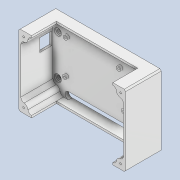
# Autodesk Inventor part: 10-06-009
Saved by Autodesk Inventor 2020 (Build 240168000, 168)
## iProperties
Created: 2019-11-09
Part Number: 10-06-009
Material: ABS Plastic
Document SubType Name: Modeling
Designer: iuliu
Density: 1.06 g/cm^3
Appearance: Smooth - White
Mass: 128.602 g
Surface Area: 588.497 cm^2
Volume: 121.322 cm^3
Description: Cutie Arduino
Author: iuliu
Subject: 027
Autodesk Inventor part; units mm, degrees
ref_plane "YZ Plane" through (0, 0, 0) normal (1, 0, 0) x (0, 1, 0)
ref_plane "XZ Plane" through (0, 0, 0) normal (0, 1, 0) x (-1, 0, 0)
ref_plane "XY Plane" through (0, 0, 0) normal (0, 0, 1) x (1, 0, 0)
sketch "Sketch1" plane through (0, 0, 0) normal (0, 0, 1) x (1, 0, 0)
  line L0 (-75, 50) -> (75, 50)
  line L1 (75, 50) -> (75, -50)
  line L2 (75, -50) -> (-75, -50)
  line L3 (-75, -50) -> (-75, 50)
  point P0 (0, 0)
  point P1 (-75, 0)
  point P2 (0, 50)
  dimension "d0" = 150
  dimension "d1" = 100
  constraints: 8 end point, 2 midpoint, 2 parallel, 1 horizontal, 1 horizontal alignment, 1 perpendicular, 1 vertical alignment
  measures "d0" distance of L0.start L0.end
  measures "d1" distance of L2.end L0.start
extrude "Extrusion1" add sketch "Sketch1" along normal blind 50
sketch "Sketch2" plane through (0, 0, 50) normal (0, 0, 1) x (1, 0, 0)
  line L0 (-33.0476, 12.9868) -> (-30.2047, 12.9868) construction
  line L1 (-30.2047, 12.9868) -> (-30.2047, 9.9388) construction
  line L2 (-30.2047, 9.9388) -> (-33.0476, 9.9388) construction
  line L3 (-33.0476, 9.9388) -> (-33.0476, 12.9868) construction
  point P0 (0, 0)
  constraints: 2 other
sketch "Sketch3" plane through (0, 0, 50) normal (0, 0, 1) x (1, 0, 0)
  line L0 (75, -50) -> (75, 50) projected
  line L1 (75, 50) -> (-75, 50) projected
  line L2 (-75, 50) -> (-75, -50) projected
  line L3 (-75, -50) -> (75, -50) projected
  line L4 (-72, 47) -> (72, 47)
  line L5 (72, 47) -> (72, -47)
  line L6 (72, -47) -> (-72, -47)
  line L7 (-72, -47) -> (-72, 47)
  point P0 (0, 0)
  dimension "d4" = 3
  constraints: 8 end point, 3 other
  measures "d4" distance between parallel lines of L1 L4
extrude "Extrusion2" cut sketch "Sketch3" against normal blind 45 contours L4 L5 L6 L7
sketch "Sketch4" plane through (-75, -50, 0) normal (-1, 0, 0) x (0, 0, 1)
  line L0 (26.325, 30.96) -> (27.325, 30.96) construction
  line L1 (27.325, 30.96) -> (27.325, 29.96) construction
  line L2 (27.325, 29.96) -> (26.325, 29.96) construction
  line L3 (26.325, 29.96) -> (26.325, 30.96) construction
  line L4 (21, 20) -> (21, 81.7649) construction
  line L5 (21, 81.7649) -> (23, 81.7649) construction
  line L6 (23, 81.7649) -> (23, 44.32) construction
  line L7 (23, 44.32) -> (31.5, 44.32) construction
  line L8 (31.5, 44.32) -> (31.5, 44.16) construction
  line L9 (31.5, 44.16) -> (31.1, 44.16) construction
  line L10 (31.1, 44.16) -> (31.1, 22) construction
  line L11 (31.1, 22) -> (23, 22) construction
  line L12 (23, 22) -> (23, 20) construction
  line L13 (23, 20) -> (21, 20) construction
  line L14 (6.5168, 74.0273) -> (6.48, 74.0735) construction
  line L15 (6.48, 74.0735) -> (6.48, 74.4839) construction
  line L16 (6.48, 74.4839) -> (7.0709, 74.9548) construction
  arc A0 (8, 75.2183) -> (7.0709, 74.9548) centre (7.85, 73.9773) ccw construction
  line L17 (8, 75.2183) -> (8, 81.2973) construction
  line L18 (8, 81.2973) -> (10, 81.2973) construction
  line L19 (10, 81.2973) -> (10, 73.7973) construction
  line L20 (10, 73.7973) -> (20.5, 73.7973) construction
  line L21 (20.5, 73.7973) -> (20.5, 61.7973) construction
  line L22 (20.5, 61.7973) -> (10, 61.7973) construction
  line L23 (10, 61.7973) -> (10, 43.2973) construction
  line L24 (10, 43.2973) -> (16.35, 43.2973) construction
  line L25 (16.35, 43.2973) -> (16.35, 42.7893) construction
  arc A1 (16.35, 34.6613) -> (16.35, 42.7893) centre (16.35, 38.7253) ccw construction
  line L26 (16.35, 34.6613) -> (16.35, 34.1533) construction
  line L27 (16.35, 34.1533) -> (10, 34.1533) construction
  line L28 (10, 34.1533) -> (10, 28.1327) construction
  line L29 (10, 28.1327) -> (8, 28.1327) construction
  line L30 (8, 28.1327) -> (8, 60.3763) construction
  arc A2 (7.0709, 60.6398) -> (8, 60.3763) centre (7.85, 61.6173) ccw construction
  line L31 (7.0709, 60.6398) -> (6.48, 61.1107) construction
  line L32 (6.48, 61.1107) -> (6.48, 61.5211) construction
  line L33 (6.48, 61.5211) -> (6.5168, 61.5673) construction
  line L34 (6.5168, 61.5673) -> (7.3078, 60.9369) construction
  arc A3 (7.3078, 60.9369) -> (8, 60.7603) centre (7.85, 61.6173) ccw construction
  line L35 (8, 60.7603) -> (8, 74.8343) construction
  arc A4 (8, 74.8343) -> (7.3078, 74.6577) centre (7.85, 73.9773) ccw construction
  line L36 (7.3078, 74.6577) -> (6.5168, 74.0273) construction
  circle A5 centre (16.35, 38.7253) radius 3.048 construction
  circle A6 centre (16.35, 38.7253) radius 1 construction
  line L37 (27.325, 41.12) -> (27.325, 40.12) construction
  line L38 (27.325, 40.12) -> (26.325, 40.12) construction
  line L39 (26.325, 40.12) -> (26.325, 41.12) construction
  line L40 (26.325, 41.12) -> (27.325, 41.12) construction
  arc A7 (24.7, 32.705) -> (24.7, 28.215) centre (27.05, 30.46) ccw construction
  line L41 (24.7, 28.215) -> (24.7, 27.625) construction
  arc A8 (24.7, 27.625) -> (24.7, 23.135) centre (27.05, 25.38) ccw construction
  line L42 (24.7, 23.135) -> (24.7, 22.78) construction
  line L43 (24.7, 22.78) -> (30.05, 22.78) construction
  line L44 (30.05, 22.78) -> (30.05, 43.22) construction
  line L45 (30.05, 43.22) -> (24.7, 43.22) construction
  line L46 (24.7, 43.22) -> (24.7, 42.865) construction
  arc A9 (24.7, 42.865) -> (24.7, 38.375) centre (27.05, 40.62) ccw construction
  line L47 (24.7, 38.375) -> (24.7, 37.785) construction
  arc A10 (24.7, 37.785) -> (24.7, 33.295) centre (27.05, 35.54) ccw construction
  line L48 (24.7, 33.295) -> (24.7, 32.705) construction
  line L49 (26.325, 24.88) -> (26.325, 25.88) construction
  line L50 (26.325, 25.88) -> (27.325, 25.88) construction
  line L51 (27.325, 25.88) -> (27.325, 24.88) construction
  line L52 (27.325, 24.88) -> (26.325, 24.88) construction
  line L53 (26.325, 35.04) -> (26.325, 36.04) construction
  line L54 (26.325, 36.04) -> (27.325, 36.04) construction
  line L55 (27.325, 36.04) -> (27.325, 35.04) construction
  line L56 (27.325, 35.04) -> (26.325, 35.04) construction
  line L57 (34.1, 47.32) -> (18, 47.32)
  line L58 (18, 47.32) -> (18, 17)
  line L59 (18, 17) -> (34.1, 17)
  line L60 (34.1, 17) -> (34.1, 47.32)
  line L61 (23.5, 76.7973) -> (7, 76.7973)
  line L62 (7, 76.7973) -> (7, 58.7973)
  line L63 (7, 58.7973) -> (23.5, 58.7973)
  line L64 (23.5, 58.7973) -> (23.5, 76.7973)
  point P0 (0, 50)
  dimension "d9" = 3
  dimension "d10" = 3
  dimension "d11" = 3
  dimension "d12" = 3
  dimension "d13" = 3
  dimension "d14" = 3
  dimension "d16" = 3
  dimension "d17" = 3
  constraints: 130 end point, 26 vertical, 23 horizontal, 18 point on circle, 11 centre point, 4 parallel, 2 perpendicular, 98 other
  measures "d9" distance from line of L10.end L60
  measures "d10" distance from line of L4.start L59
  measures "d11" distance from line of L6.end L57
  measures "d12" distance from line of L58 L4.start
  measures "d13" distance from line of L21.end L64
  measures "d14" distance from line of L22.end L63
  measures "d16" distance from line of L19.end L61
  measures "d17" distance from line of L62 L19.end
extrude "Extrusion3" cut sketch "Sketch4" against normal up to surface (3 mm away) contours L64 L63 L62 L61
sketch "Sketch5" plane through (-75, 50, 0) normal (0, 1, 0) x (1, 0, 0)
  circle A0 centre (112.5, -25) radius 7.5
  circle A1 centre (37.5, -25) radius 7.5
  circle A2 centre (75, -25) radius 7.5
  line L0 (150, 0) -> (150, -50) projected
  line L1 (0, 0) -> (0, -50) projected
  point P0 (75, 0)
  point P1 (0, -25)
  point P2 (0, -25)
  dimension "d20" = 15
  dimension "d21" = 15
  dimension "d22" = 15
  dimension "d23" = 37.5
  dimension "d24" = 37.5
  dimension "d25" = 37.5
  constraints: 3 centre point, 3 horizontal alignment, 2 midpoint
  measures "d20" diameter of A0
  measures "d21" diameter of A1
  measures "d22" diameter of A2
  measures "d23" distance from line of L0 A0.centre
  measures "d24" distance of A2.centre A0.centre
  measures "d25" distance of A2.centre A1.centre
extrude "Extrusion4" [suppressed]
sketch "Sketch6" plane through (0, 0, 5) normal (0, 0, 1) x (1, 0, 0)
  line L0 (-68, -43) -> (68, -43) construction
  line L1 (68, -43) -> (68, 43) construction
  line L2 (68, 43) -> (-68, 43) construction
  line L3 (-68, 43) -> (-68, -43) construction
  line L4 (-72, -47) -> (-72, 47) projected
  line L5 (-72, 47) -> (72, 47) projected
  line L6 (72, 47) -> (72, -47) projected
  line L7 (72, -47) -> (-72, -47) projected
  point P0 (0, 0)
  dimension "d28" = 4
  dimension "d29" = 4
  dimension "d30" = 4
  dimension "d31" = 4
  constraints: 8 end point, 2 parallel, 1 horizontal, 1 perpendicular
  measures "d28" distance between parallel lines of L3 L4
  measures "d29" distance between parallel lines of L5 L2
  measures "d30" distance between parallel lines of L6 L1
  measures "d31" distance between parallel lines of L7 L0
hole "Hole1" at (-68, -43, 5) at (-68, 43, 5) at (68, -43, 5) at (68, 43, 5) direction (0, 0, -1) diameter 2.5 end through all
sketch "Sketch7" plane through (0, 0, 5) normal (0, 0, 1) x (1, 0, 0)
  circle A0 centre (-68, -43) radius 1.25 projected
  circle A1 centre (-68, 43) radius 1.25 projected
  circle A2 centre (68, 43) radius 1.25 projected
  circle A3 centre (68, -43) radius 1.25 projected
  circle A4 centre (-68, -43) radius 6
  circle A5 centre (-68, 43) radius 6
  circle A6 centre (68, -43) radius 6
  circle A7 centre (68, 43) radius 6
  point P0 (0, 0)
  dimension "d39" = 12
  constraints: 4 centre point, 4 coincident, 3 equal radius
  measures "d39" diameter of A4
extrude "Extrusion5" add sketch "Sketch7" along normal up to surface (45 mm away)
fillet "Fillet1" radius 5 8 edges at (-72, 38.5279, 27.5) (-63.5279, 47, 27.5) (-63.5279, -47, 27.5) (-72, -38.5279, 27.5) (63.5279, 47, 27.5) (63.5279, -47, 27.5) (72, 38.5279, 27.5) (72, -38.5279, 27.5)
sketch "Sketch10" plane through (0, 0, 0) normal (0, 0, -1) x (-1, 0, 0)
  line L0 (-75, 50) -> (-55, 50)
  line L1 (-55, 50) -> (-55, -50)
  line L2 (-55, -50) -> (-75, -50)
  line L3 (-75, -50) -> (-75, 50)
  line L4 (-75, 50) -> (75, 50) projected
  line L5 (75, -50) -> (-75, -50) projected
  line L6 (-75, -50) -> (-75, 50) projected
  point P0 (0, 0)
  dimension "d46" = 20
  constraints: 8 end point, 3 collinear, 2 parallel, 1 horizontal, 1 perpendicular
  measures "d46" distance of L0.start L0.end
extrude "Extrusion7" [suppressed]
sketch "Sketch11" plane through (0, 0, 5) normal (0, 0, 1) x (1, 0, 0)
  line L0 (72, 32.0455) -> (72, -32.0455) projected
  line L1 (57.0455, -47) -> (-57.0455, -47) projected
  line L2 (75, 50) -> (-75, 50) projected
  point P0 (0, 0)
  point P1 (65, -17)
  point P2 (65, 20)
  dimension "d49" = 7
  dimension "d50" = 30
  dimension "d51" = 30
  constraints: 1 vertical alignment
  measures "d49" distance from line of L0 point (65, -17)
  measures "d50" distance from line of L1 point (65, -17)
  measures "d51" distance from line of L2 point (65, 20)
hole "Hole2" at (65, -17, 5) at (65, 20, 5) direction (0, 0, -1) diameter 7 end through all
sketch "Sketch12" plane through (0, 0, 5) normal (0, 0, 1) x (1, 0, 0)
  line L0 (-50, -42) -> (50, -42) construction
  line L1 (-50, -47) -> (50, -47)
  line L2 (50, -37) -> (-50, -37)
  arc A0 (-50, -37) -> (-50, -47) centre (-50, -42) ccw
  arc A1 (50, -47) -> (50, -37) centre (50, -42) ccw
  line L3 (-66.4643, 0) -> (-31.6341, 0) construction
  line L4 (57.0455, -47) -> (-57.0455, -47) construction
  line L5 (-50, 47) -> (50, 47)
  line L6 (50, 37) -> (-50, 37)
  arc A2 (-50, 47) -> (-50, 37) centre (-50, 42) ccw
  arc A3 (50, 37) -> (50, 47) centre (50, 42) ccw
  point P0 (0, 0)
  point P1 (0, -42)
  point P2 (-49.0492, 0)
  dimension "d59" = 10
  dimension "d60" = 5
  dimension "d61" = 100
  constraints: 14 end point, 8 point on circle, 6 symmetric about line, 4 centre point, 4 tangent, 2 horizontal, 2 midpoint, 1 horizontal alignment, 1 parallel, 1 vertical alignment, 2 other
  measures "d59" distance between parallel lines of L2 L1
  measures "d60" distance between parallel lines of L4 L0
  measures "d61" distance of L0.start L0.end
extrude "Extrusion8" cut sketch "Sketch12" against normal through all
sketch "Sketch13" plane through (0, 0, 5) normal (0, 0, 1) x (1, 0, 0)
  circle A0 centre (-53, -19.3673) radius 1.6078 construction
  circle A1 centre (-51.7238, 29.1287) radius 1.6078 construction
  circle A2 centre (22.9611, 28.7987) radius 1.6 construction
  circle A3 centre (29.9537, -19.3673) radius 1.6078 construction
  circle A4 centre (-63.3989, 10.0987) radius 1.1 construction
  point P0 (0, 0)
hole "Hole3" at (-53, -19.3673, 5) at (-51.7238, 29.1287, 5) at (29.9537, -19.3673, 5) at (22.9611, 28.7987, 5) direction (0, 0, -1) diameter 2.459 end through all thread size "M3x0.5" class "6H" standard "ISO Metric profile"
chamfer "Chamfer1" distance 2 angle 45 4 edges at (-53, -18.1378, 0) (29.9537, -18.1378, 0) (-51.7238, 30.3582, 0) (22.9611, 30.0282, 0)
sketch "Sketch14" plane through (0, 0, 5) normal (0, 0, 1) x (1, 0, 0)
  circle A0 centre (-68, -43) radius 1.25 projected
  circle A1 centre (-68, 43) radius 1.25 projected
  line L0 (-75, 50) -> (-75, -50) projected
  point P0 (0, 0)
  point P1 (-65, -28)
  point P2 (-65, 28)
  dimension "d74" = 15
  dimension "d75" = 15
  dimension "d83" = 10
  constraints: 1 vertical alignment
  measures "d74" vertical distance of A0.centre point (-65, -28)
  measures "d75" vertical distance of A1.centre point (-65, 28)
  measures "d83" distance from line of point (-65, -28) L0
hole "Hole4" at (-65, -28, 5) at (-65, 28, 5) direction (0, 0, -1) diameter 5 end through all counterbore diameter 10 counterbore depth 2
sketch "Sketch15" plane through (-75, 50, 50) normal (0, 1, 0) x (1, 0, 0)
  line L0 (125, 5) -> (25, 5) construction
  line L1 (125, 3.5) -> (25, 3.5)
  line L2 (25, 6.5) -> (125, 6.5)
  arc A0 (125, 3.5) -> (125, 6.5) centre (125, 5) ccw
  arc A1 (25, 6.5) -> (25, 3.5) centre (25, 5) ccw
  line L3 (0, 50) -> (0, 0) projected
  line L4 (150, 50) -> (150, 0) projected
  line L5 (150, 0) -> (0, 0) projected
  point P0 (75, 50)
  point P1 (75, 5)
  point P2 (150, 70)
  dimension "d84" = 3
  dimension "d85" = 25
  dimension "d86" = 25
  dimension "d87" = 5
  constraints: 8 end point, 4 point on circle, 4 tangent, 2 centre point, 1 horizontal, 1 midpoint, 1 parallel
  measures "d84" distance between parallel lines of L2 L1
  measures "d85" distance from line of L3 L0.end
  measures "d86" distance from line of L4 L0.start
  measures "d87" distance between parallel lines of L0 L5
extrude "Extrusion9" [suppressed]
pattern_linear "Rectangular Pattern1" [suppressed]
sketch "Sketch16" plane through (0, 0, 0) normal (0, 1, 0) x (-1, 0, 0)
  line L0 (57.0455, 50) -> (57.0455, 5) projected
  line L1 (-57.0455, 5) -> (-57.0455, 50) projected
  line L2 (50, 5) -> (-50, 5) projected
  line L3 (-57.0455, 50) -> (-57.0455, 5) projected
  line L4 (-57.0455, 15) -> (57.0455, 15)
  line L5 (57.0455, 5) -> (57.0455, 50) projected
  line L6 (-57.0455, 50) -> (57.0455, 50)
  line L7 (75, 50) -> (-75, 50) projected
  point P0 (0, 0)
  dimension "d93" = 10
  constraints: 4 end point, 2 point on line, 1 collinear, 1 perpendicular
  measures "d93" distance between parallel lines of L2 L4
extrude "Extrusion10" cut sketch "Sketch16" against normal through all both and the other way through all
chamfer "Chamfer2" distance 2 angle 45 4 edges at (75, 50, 25) (-75, 50, 25) (-75, -50, 25) (75, -50, 25)
sketch "Sketch17" plane through (0, 0, 5) normal (0, 0, 1) x (1, 0, 0)
  circle A0 centre (-65, -28) radius 5 projected
  circle A1 centre (-65, 28) radius 5 projected
  circle A2 centre (29.9537, -19.3673) radius 1.2295 projected
  circle A3 centre (-53, -19.3673) radius 1.2295 projected
  circle A4 centre (-51.7238, 29.1287) radius 1.2295 projected
  circle A5 centre (22.9611, 28.7987) radius 1.2295 projected
  arc A6 (50, 37) -> (50, 47) centre (50, 42) ccw projected
  line L0 (50, 37) -> (-50, 37) projected
  arc A7 (-50, 47) -> (-50, 37) centre (-50, 42) ccw projected
  line L1 (-57.0455, 47) -> (-50, 47) projected
  arc A8 (-57.0455, 47) -> (-62.0248, 42.4545) centre (-57.0455, 42) ccw projected
  arc A9 (-67.4545, 37.0248) -> (-62.0248, 42.4545) centre (-68, 43) ccw projected
  arc A10 (-67.4545, 37.0248) -> (-72, 32.0455) centre (-67, 32.0455) ccw projected
  line L2 (-72, -32.0455) -> (-72, 32.0455) projected
  arc A11 (-72, -32.0455) -> (-67.4545, -37.0248) centre (-67, -32.0455) ccw projected
  arc A12 (-62.0248, -42.4545) -> (-67.4545, -37.0248) centre (-68, -43) ccw projected
  arc A13 (-62.0248, -42.4545) -> (-57.0455, -47) centre (-57.0455, -42) ccw projected
  line L3 (-50, -47) -> (-57.0455, -47) projected
  arc A14 (-50, -37) -> (-50, -47) centre (-50, -42) ccw projected
  line L4 (-50, -37) -> (50, -37) projected
  arc A15 (50, -47) -> (50, -37) centre (50, -42) ccw projected
  line L5 (57.0455, -47) -> (50, -47) projected
  arc A16 (57.0455, -47) -> (62.0248, -42.4545) centre (57.0455, -42) ccw projected
  arc A17 (67.4545, -37.0248) -> (62.0248, -42.4545) centre (68, -43) ccw projected
  arc A18 (67.4545, -37.0248) -> (72, -32.0455) centre (67, -32.0455) ccw projected
  line L6 (72, 32.0455) -> (72, -32.0455) projected
  arc A19 (72, 32.0455) -> (67.4545, 37.0248) centre (67, 32.0455) ccw projected
  arc A20 (62.0248, 42.4545) -> (67.4545, 37.0248) centre (68, 43) ccw projected
  arc A21 (62.0248, 42.4545) -> (57.0455, 47) centre (57.0455, 42) ccw projected
  line L7 (50, 47) -> (57.0455, 47) projected
  circle A22 centre (65, 20) radius 3.5 projected
  circle A23 centre (65, -17) radius 3.5 projected
  circle A24 centre (-51.7238, 29.1287) radius 1.2295 projected
  circle A25 centre (-51.7238, 29.1287) radius 3
  circle A26 centre (22.9611, 28.7987) radius 1.2295 projected
  circle A27 centre (22.9611, 28.7987) radius 3.2295
  circle A28 centre (29.9537, -19.3673) radius 3.2295
  circle A29 centre (-53, -19.3673) radius 3
  circle A30 centre (-51.7238, 29.1287) radius 3.2295 projected
  point P0 (0, 0)
  dimension "d99" = 6
  constraints: 4 centre point, 3 coincident, 3 equal radius, 1 concentric
  measures "d99" diameter of A25
extrude "Extrusion11" add sketch "Sketch17" along normal blind 3 contours A25 | A27 | A28 | A29
body "Solid1"
